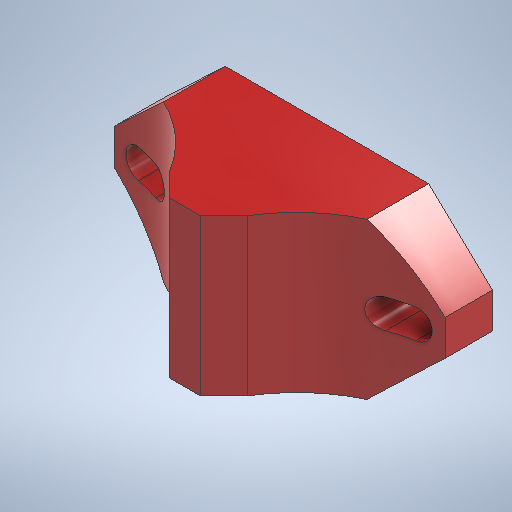
# Autodesk Inventor part: scanner
Saved by Autodesk Inventor 2025.1 (Build 291241000, 241)
## iProperties
Created: 2025-02-14
Part Number: scanner
Material: Generic
Document SubType Name: Modeling
Designer: m_kni
Density: 1 g/cm^3
Appearance: Default
Author: m_kni
Autodesk Inventor part; units mm, degrees
ref_plane "YZ Plane" through (0, 0, 0) normal (1, 0, 0) x (0, 1, 0)
ref_plane "XZ Plane" through (0, 0, 0) normal (0, 1, 0) x (-1, 0, 0)
ref_plane "XY Plane" through (0, 0, 0) normal (0, 0, 1) x (1, 0, 0)
sketch "Sketch1" plane through (0, 0, 0) normal (0, 0, 1) x (1, 0, 0)
  line L0 (35, -3.75) -> (-35, -3.75)
  line L1 (-35, -3.75) -> (-35, 3.75)
  line L2 (-35, 3.75) -> (35, 3.75)
  line L3 (35, 3.75) -> (35, -3.75)
  line L4 (35, -3.75) -> (-35, 3.75) construction
  line L5 (-35, -3.75) -> (35, 3.75) construction
  line L6 (21.5, -16.5) -> (-21.5, -16.5)
  line L7 (-21.5, -16.5) -> (-21.5, 16.5)
  line L8 (-21.5, 16.5) -> (21.5, 16.5)
  line L9 (21.5, 16.5) -> (21.5, -16.5)
  line L10 (21.5, -16.5) -> (-21.5, 16.5) construction
  line L11 (-21.5, -16.5) -> (21.5, 16.5) construction
  line L12 (-35, -3.75) -> (-21.5, -16.5)
  line L13 (-35, 3.75) -> (-21.5, 16.5)
  arc A0 (32.3113, 4.5234) -> (35, 3.75) centre (34.605, 7.4371) ccw
  line L14 (21.5, -16.5) -> (35, -3.75)
  line L15 (35, 3.75) -> (21.5, 16.5)
  point P0 (0, 0)
  dimension "d0" = 70
  dimension "d1" = 7.5
  dimension "d2" = 43
  dimension "d3" = 33
  constraints: 32 end point, 4 midpoint, 4 parallel, 2 horizontal, 2 perpendicular, 2 point on circle, 1 centre point, 1 tangent
  measures "d0" distance of L1.end L2.end
  measures "d1" distance of L0.end L1.end
  measures "d2" distance of L7.end L8.end
  measures "d3" distance of L6.end L7.end
extrude "Extrusion1" add sketch "Sketch1" along normal blind 30
sketch "Sketch2" plane through (-21.5, -16.5, 0) normal (0, -1, 0) x (1, 0, 0)
  line L0 (43, 30) -> (0, 30) projected
  line L1 (43, 0) -> (0, 0) projected
  line L2 (0, 30) -> (43, 30)
  line L3 (43, 30) -> (43, 0)
  line L4 (43, 0) -> (0, 0)
  line L5 (0, 0) -> (0, 30)
  line L6 (21.5, 30) -> (24.75, 30)
  line L7 (56.5, 0) -> (56.5, 30) projected
  line L8 (56.5, 0) -> (56.5, 10)
  line L9 (24.75, 30) -> (29.6997, 25.0503)
  arc A0 (29.6997, 25.0503) -> (56.5, 10) centre (56.5, 41.387) ccw
  arc A1 (55.355, 10.0209) -> (56.5, 10) centre (56.5, 41.387) ccw
  line L10 (56.5, 10) -> (46.9475, 10)
  line L11 (21.5, 30) -> (21.5, 26.75)
  line L12 (21.5, 30) -> (18.25, 30)
  line L13 (-13.5, 0) -> (-13.5, 30)
  line L14 (18.25, 30) -> (13.3003, 25.0503)
  arc A2 (-13.5, 10) -> (13.3003, 25.0503) centre (-13.5, 41.387) ccw
  line L15 (43, 30) -> (56.5, 30) projected
  line L16 (43, 0) -> (43, 30) projected
  line L17 (56.5, 30) -> (43, 30) projected
  line L18 (43, 0) -> (43, 30) projected
  line L19 (56.5, 0) -> (43, 0) projected
  line L20 (56.5, 0) -> (56.5, 30) projected
  line L21 (43, 0) -> (56.5, 0) projected
  line L22 (43, 0) -> (56.5, 0) projected
  line L23 (56.5, 0) -> (56.5, 30) projected
  line L24 (43, 30) -> (56.5, 30) projected
  line L25 (43, 0) -> (43, 30) projected
  line L26 (56.5, 0) -> (56.5, 30) projected
  line L27 (56.5, 0) -> (56.5, 30) projected
  line L28 (56.5, 0) -> (43, 0) projected
  line L29 (43, 0) -> (43, 30) projected
  line L30 (56.5, 30) -> (43, 30) projected
  line L31 (56.5, 0) -> (56.5, 30) projected
  line L32 (43, 0) -> (56.5, 0) projected
  line L33 (0, 0) -> (43, 0) projected
  line L34 (-13.5, 0) -> (0, 0) projected
  line L35 (0, 0) -> (-13.5, 0) projected
  line L36 (43, 0) -> (0, 0) projected
  line L37 (56.5, 0) -> (43, 0) projected
  line L38 (43, 30) -> (56.5, 30) projected
  line L39 (56.5, 30) -> (43, 30) projected
  line L40 (43, 30) -> (0, 30) projected
  line L41 (0, 30) -> (-13.5, 30) projected
  line L42 (-13.5, 30) -> (0, 30) projected
  line L43 (0, 30) -> (43, 30) projected
  line L44 (0, 30) -> (43, 30) projected
  line L45 (0, 0) -> (43, 0) projected
  line L46 (43, 0) -> (0, 0) projected
  line L47 (0, 0) -> (0, 30) projected
  line L48 (43, 30) -> (0, 30) projected
  line L49 (43, 0) -> (43, 30) projected
  line L50 (0, 0) -> (43, 0) projected
  line L51 (43, 0) -> (43, 30) projected
  line L52 (0, 30) -> (43, 30) projected
  line L53 (0, 0) -> (0, 30) projected
  line L54 (0, 0) -> (0, 30) projected
  line L55 (0, 0) -> (0, 30) projected
  line L56 (0, 0) -> (-13.5, 0) projected
  line L57 (-13.5, 0) -> (-13.5, 30) projected
  line L58 (-13.5, 0) -> (-13.5, 30) projected
  line L59 (-13.5, 0) -> (0, 0) projected
  line L60 (0, 0) -> (-13.5, 0) projected
  line L61 (-13.5, 0) -> (-13.5, 30) projected
  line L62 (0, 30) -> (-13.5, 30) projected
  line L63 (0, 0) -> (0, 30) projected
  line L64 (-13.5, 0) -> (-13.5, 30) projected
  line L65 (-13.5, 0) -> (-13.5, 30) projected
  line L66 (-13.5, 0) -> (0, 0) projected
  line L67 (0, 0) -> (0, 30) projected
  line L68 (-13.5, 30) -> (0, 30) projected
  line L69 (-13.5, 0) -> (-13.5, 30) projected
  line L70 (-13.5, 30) -> (0, 30) projected
  line L71 (0, 30) -> (-13.5, 30) projected
  point P0 (21.5, 0)
  dimension "d6" = 3.25
  dimension "d7" = 10
  dimension "d8" = 7
  dimension "d9" = 45
  constraints: 24 end point, 7 point on circle, 6 symmetric about line, 3 centre point, 3 point on line, 2 horizontal, 2 parallel, 2 tangent, 1 concentric, 1 midpoint, 1 perpendicular, 1 vertical, 9 other
  measures "d6" distance of L6.start L6.end
  measures "d7" distance of L7.start L8.end
  measures "d8" distance of L6.end L9.end
  measures "d9" angle of L0 L9
extrude "Extrusion2" cut sketch "Sketch2" against normal blind 36.35 contours L3 A0 L9 L0 | L15 L7 A0 L3 | L14 A2 L5 L0 | L5 A2 L13 L41
sketch "Sketch3" plane through (0, 0, 0) normal (0, 0, -1) x (-1, 0, 0)
  line L0 (35, 3.75) -> (35, -3.75) projected
  circle A0 centre (29.3, 0) radius 3.1
  line L1 (32.4, 0) -> (24.3, 0)
  circle A1 centre (24.3, 0) radius 3.1
  line L2 (29.3, -3.1) -> (24.3, -3.1)
  line L3 (29.3, 3.1) -> (24.3, 3.1)
  line L4 (0, 0) -> (0, -2.435)
  circle A2 centre (-29.3, 0) radius 3.1
  line L5 (-32.4, 0) -> (-24.3, 0)
  circle A3 centre (-24.3, 0) radius 3.1
  line L6 (-29.3, -3.1) -> (-24.3, -3.1)
  line L7 (-29.3, 3.1) -> (-24.3, 3.1)
  dimension "d12" = 5.7
  dimension "d13" = 6.2
  dimension "d14" = 8.1
  dimension "d15" = 6.2
  constraints: 14 end point, 10 point on circle, 9 symmetric about line, 4 centre point, 4 coincident, 2 tangent, 1 horizontal, 1 vertical, 2 other
  measures "d12" distance from line of point (29.3, 0) L0
  measures "d13" diameter of A0
  measures "d14" distance of L1.start L1.end
  measures "d15" diameter of A1
extrude "Extrusion3" cut sketch "Sketch3" against normal blind 36.35
body "Solid1"
